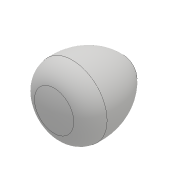
# Autodesk Inventor part: shell_front
Saved by Autodesk Inventor 2017 (Build 210142000, 142)
## iProperties
Created: 2018-06-30
Part Number: shell_front
Material: Generic
Document SubType Name: Modeling
Designer: mfans
Density: 1 g/cm^3
Appearance: Default
Author: mfans
Autodesk Inventor part; units mm, degrees
ref_plane "YZ Plane" through (0, 0, 0) normal (1, 0, 0) x (0, 1, 0)
ref_plane "XZ Plane" through (0, 0, 0) normal (0, 1, 0) x (-1, 0, 0)
ref_plane "XY Plane" through (0, 0, 0) normal (0, 0, 1) x (1, 0, 0)
sketch "Sketch1" plane through (0, 0, 0) normal (0, 0, 1) x (1, 0, 0)
  line L0 (0, 0) -> (32, 0)
  line L1 (0, 0) -> (-32, 0)
  arc A0 (0, -6.6788) -> (32, 0) centre (0, 73.3212) ccw
  arc A1 (32, 0) -> (7.0818, 69.3212) centre (-26.5172, 18.1046) ccw
  line L2 (0, 69.3212) -> (0, -6.6788)
  line L3 (0, 69.3212) -> (7.0818, 69.3212)
  dimension "d0" = 32
  dimension "d1" = 32
  dimension "d2" = 80
  dimension "d3" = 4
  constraints: 8 end point, 4 point on circle, 3 horizontal, 2 centre point
  measures "d0" distance of L0.start L0.end
  measures "d1" distance of L0.start L1.end
  measures "d2" radius of A0
  measures "d3" distance from line of A0.centre L3
revolve "Revolution1" add sketch "Sketch1" angle 360 about axis through (0, 69.3212, 0) along (0, -1, 0)
fillet "Fillet1" radius 20 1 edges at (-32, 0, 0)
fillet "Fillet2" radius 20 1 edges at (-7.0818, 69.3212, 0)
body "Solid1"
